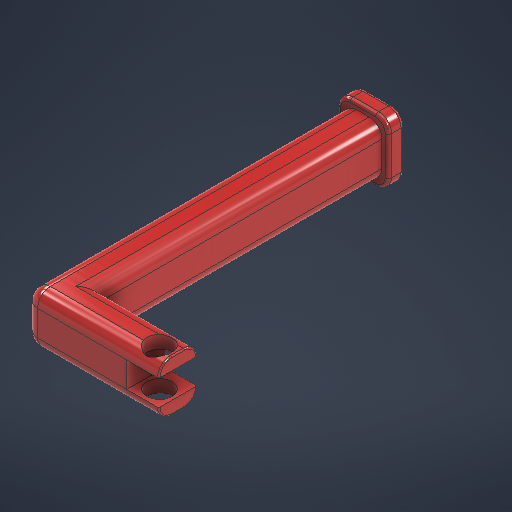
# Autodesk Inventor part: Part3final
Saved by Autodesk Inventor 2026 (Build 300175050, 175E)
## iProperties
Created: 2026-05-04
Part Number: Part3final
Material: Steel, Carbon
Document SubType Name: Modeling
Designer: ptp527
Mass: 22840.5 g
Surface Area: 1825.2 cm^2
Volume: 2909.62 cm^3
Density: 7.85 g/cm^3
Appearance: Semi-Polished
Author: ptp527
Autodesk Inventor part; units mm, degrees
ref_plane "YZ Plane" through (0, 0, 0) normal (1, 0, 0) x (0, 1, 0)
ref_plane "XZ Plane" through (0, 0, 0) normal (0, 1, 0) x (-1, 0, 0)
ref_plane "XY Plane" through (0, 0, 0) normal (0, 0, 1) x (1, 0, 0)
sketch "Sketch1" plane through (0, 0, 0) normal (0, 0, 1) x (1, 0, 0)
  line L0 (-30, -40) -> (30, -40)
  line L1 (30, -40) -> (30, 40)
  line L2 (30, 40) -> (-30, 40)
  line L3 (-30, 40) -> (-30, -40)
  line L4 (-30, -40) -> (30, 40) construction
  line L5 (30, -40) -> (-30, 40) construction
  point P0 (0, 0)
  dimension "d0" = 80
  dimension "d1" = 60
  constraints: 12 end point, 2 midpoint, 2 parallel, 1 horizontal, 1 perpendicular
  measures "d0" distance of L2.end L0.start
  measures "d1" distance of L1.end L2.end
extrude "Extrusion1" add sketch "Sketch1" along normal blind 500
sketch "Sketch2" plane through (30, -40, 0) normal (1, 0, 0) x (0, 0, -1)
  line L0 (-500, 0) -> (-500, 80) projected
  line L1 (-440, 0) -> (-500, 0)
  line L2 (-500, 0) -> (-500, 80)
  line L3 (-500, 80) -> (-440, 80)
  line L4 (-440, 80) -> (-440, 0)
  line L5 (-440, 0) -> (-500, 80) construction
  line L6 (-500, 0) -> (-440, 80) construction
  point P0 (0, 40)
  point P1 (-470, 40)
  point P2 (-440, 40)
  point P3 (-500, 40)
  dimension "d4" = 30
  dimension "d5" = 30
  dimension "d6" = 30
  dimension "d7" = 40
  dimension "d8" = 40
  constraints: 12 end point, 4 midpoint, 2 parallel, 1 horizontal, 1 perpendicular
  measures "d4" distance from line of L0 point (-470, 40)
  measures "d5" distance of point (-440, 40) point (-470, 40)
  measures "d6" distance of point (-500, 40) point (-470, 40)
  measures "d7" distance from line of point (-470, 40) L1
  measures "d8" distance from line of L3 point (-470, 40)
extrude "Extrusion2" add sketch "Sketch2" along normal blind 150
fillet "Fillet1" radius 20 4 edges at (30, 40, 220) (-30, 40, 250) (30, -40, 220) (-30, -40, 250)
fillet "Fillet2" radius 20 8 edges at (20, 40, 440) (85, 40, 500) (-24.1421, 34.1421, 500) (-30, 0, 500) (-24.1421, -34.1421, 500) (85, -40, 500) (105, -40, 440) (20, -40, 440)
sketch "Sketch3" plane through (0, 0, 0) normal (0, 0, -1) x (-1, 0, 0)
  line L0 (-40, -50) -> (40, -50)
  line L1 (40, -50) -> (40, 50)
  line L2 (40, 50) -> (-40, 50)
  line L3 (-40, 50) -> (-40, -50)
  line L4 (-40, -50) -> (40, 50) construction
  line L5 (40, -50) -> (-40, 50) construction
  point P0 (0, 0)
  dimension "d13" = 80
  dimension "d14" = 100
  constraints: 12 end point, 2 midpoint, 2 parallel, 1 horizontal, 1 perpendicular
  measures "d13" distance of L1.end L2.end
  measures "d14" distance of L0.end L1.end
extrude "Extrusion3" add sketch "Sketch3" along normal blind 25
fillet "Fillet3" radius 5 8 edges at (40, 0, 0) (40, 0, -25) (0, 50, 0) (0, 50, -25) (-40, 0, 0) (0, -50, 0) (0, -50, -25) (-40, 0, -25)
fillet "Fillet4" radius 20 12 edges at (40, 50, -12.5) (38.5355, 48.5355, -23.5355) (38.5355, 48.5355, -1.4645) (-40, 50, -12.5) (-38.5355, 48.5355, -23.5355) (-38.5355, 48.5355, -1.4645) (40, -50, -12.5) (38.5355, -48.5355, -23.5355) (38.5355, -48.5355, -1.4645) (-40, -50, -12.5) (-38.5355, -48.5355, -23.5355) (-38.5355, -48.5355, -1.4645)
sketch "Sketch4" plane through (180, -40, 0) normal (1, 0, 0) x (0, 0, -1)
  line L0 (-527.9087, 60) -> (-418.267, 60)
  line L1 (-418.267, 60) -> (-418.267, 20)
  line L2 (-418.267, 20) -> (-527.9087, 20)
  line L3 (-527.9087, 20) -> (-527.9087, 60)
  line L4 (-527.9087, 60) -> (-418.267, 20) construction
  line L5 (-418.267, 60) -> (-527.9087, 20) construction
  line L6 (-460, 80) -> (-480, 80) projected
  line L7 (-480, 0) -> (-460, 0) projected
  point P0 (0, 40)
  point P1 (-473.0878, 40)
  point P2 (-473.0878, 60)
  point P3 (-473.0878, 20)
  dimension "d19" = 20
  dimension "d20" = 20
  dimension "d21" = 54.8209
  dimension "d22" = 20
  dimension "d23" = 20
  constraints: 12 end point, 4 midpoint, 2 parallel, 1 horizontal, 1 perpendicular
  measures "d19" distance of point (-473.088, 60) point (-473.088, 40)
  measures "d20" distance from line of point (-473.088, 60) L6
  measures "d21" distance from line of L1 point (-473.088, 40)
  measures "d22" distance of point (-473.088, 20) point (-473.088, 40)
  measures "d23" distance from line of L7 point (-473.088, 20)
extrude "Extrusion4" cut sketch "Sketch4" against normal blind 50
sketch "Sketch5" plane through (-10, 40, 480) normal (0, 1, 0) x (1, 0, 0)
  circle A0 centre (165, 6.2634) radius 20
  line L0 (190, 20) -> (190, 0) projected
  point P0 (10, 480)
  dimension "d26" = 25
  dimension "d27" = 40
  constraints: 1 centre point
  measures "d26" distance from line of L0 A0.centre
  measures "d27" diameter of A0
extrude "Extrusion5" cut sketch "Sketch5" along normal mid plane 200
fillet "Fillet5" radius 2 6 edges at (180, 34.1421, 445.8579) (180, 40, 470) (180, 34.1421, 494.1421) (180, -40, 470) (180, -34.1421, 445.8579) (180, -34.1421, 494.1421)
body "Solid1"
